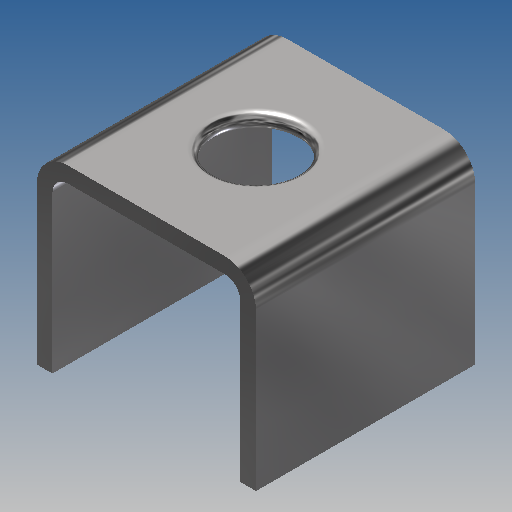
# Autodesk Inventor part: DD_KVD_002_11
Saved by Autodesk Inventor 2017.3 (Build 213256000, 256)
## iProperties
Created: 2023-11-02
Part Number: DD_KVD_002_11
Material: Nerezová ocel
Document SubType Name: Sheet Metal
Designer: Darena
Density: 8 g/cm^3
Sheet Metal Rule: Výchozí_mm
Appearance: Pololeštěná
Flat Pattern Width: 3.5 cm
Flat Pattern Length: 8.63097 cm
Flat Pattern Area: 30.2084 cm^2
Sheet Metal Width: 35,000 mm
Sheet Metal Length: 86,310 mm
Sheet Metal Area: 3020,841 mm^2
Author: Darena
Autodesk Inventor part; units mm, degrees
ref_plane "YZ Plane" through (0, 0, 0) normal (1, 0, 0) x (0, 1, 0)
ref_plane "XZ Plane" through (0, 0, 0) normal (0, 1, 0) x (-1, 0, 0)
ref_plane "XY Plane" through (0, 0, 0) normal (0, 0, 1) x (1, 0, 0)
sketch "Náčrt2" plane through (0, 0, 0) normal (0, 1, 0) x (-1, 0, 0)
  line L0 (17.5, 17.5) -> (-17.5, 17.5)
  line L1 (-17.5, 17.5) -> (-17.5, -17.5)
  line L2 (-17.5, -17.5) -> (17.5, -17.5)
  line L3 (17.5, -17.5) -> (17.5, 17.5)
  circle A0 centre (0, 0) radius 6.55
  point P0 (17.5, 0)
  point P1 (0, 17.5)
  dimension "d0" = 35
  dimension "d1" = 35
  dimension "d22" = 13.1
  constraints: 8 end point, 2 midpoint, 2 parallel, 1 centre point, 1 coincident, 1 horizontal, 1 horizontal alignment, 1 perpendicular, 1 vertical alignment
  measures "d0" distance of L0.start L0.end
  measures "d1" distance of L2.end L0.start
  measures "d22" diameter of A0
extrude "Vysunutí1" add sketch "Náčrt2" along normal blind 2.5
sketch "Náčrt5" plane through (-15, 2.5, -17.5) normal (-1, 0, 0) x (0, -1, 0)
  line L0 (0, 35) -> (0, 0)
  line L1 (0, 0) -> (30, 0)
  line L2 (30, 0) -> (30, 35)
  line L3 (30, 35) -> (0, 35)
  constraints: 6 end point, 1 horizontal, 1 perpendicular, 1 vertical
edge flange "Obruba2" height 30 angle 90 thickness 2.5 bend radius 2.5 thickness toward (-1, 0, 0) relief tear relief width 2.5 relief depth 1.25 corner gap 2.5 corner form 0 edges at (-17.5, 0, 0) (17.5, 0, 0) wall of the first edge with corners at (-15, 2.5, 17.5) (-15, 2.5, -17.5) (-15, -27.5, -17.5) (-15, -27.5, 17.5)
bend "Ohyb2"
corner "Roh2"
fillet "Zaoblení6" radius 1.25 1 edges at (6.55, 2.5, 0)
fillet "Zaoblení7" radius 1.25 1 edges at (6.55, 0, 0)
equation "\"d29\" = ŠířkaVýštipu"
equation "\"d30\" = HloubkaVýštipu"
equation "\"d31\" = MinimálníZbytek"
equation "\"d32\" = PoloměrOhybu"
equation "\"d35\" = PoloměrOhybu"
equation "\"d36\" = VelikostRohovéhoVýštipu"
equation "\"d37\" = VelikostMezery"
equation "\"d38\" = VelikostJacobihoPoloměru"
equation "\"PoloměrOhybu\" = Tloušťka"
equation "\"ŠířkaVýštipu\" = Tloušťka"
equation "\"HloubkaVýštipu\" = 0.5 * Tloušťka"
equation "\"MinimálníZbytek\" = 2 * Tloušťka"
equation "\"PřechodovýPoloměr\" = PoloměrOhybu"
equation "\"VelikostJacobihoPoloměru\" = PoloměrOhybu"
equation "\"VelikostMezery\" = Tloušťka"
equation "\"VelikostRohovéhoVýštipu\" = 10"
equation "\"Tloušťka\" = 2.5"
